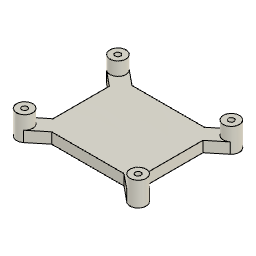
Toolhead Breakout PCB Mount (Autodesk Fusion 360 design; units mm, degrees)
Autodesk Fusion 360 part; units mm, degrees
sketch "Sketch1" plane through (0, 0, 0) normal (0, 0, 1) x (1, 0, 0)
  line L0 (21.185, 17.41) -> (-21.185, 17.41) construction
  line L1 (-21.185, 17.41) -> (-21.185, -17.41) construction
  line L2 (-21.185, -17.41) -> (21.185, -17.41) construction
  line L3 (21.185, -17.41) -> (21.185, 17.41) construction
  line L4 (21.185, 17.41) -> (-21.185, -17.41) construction
  line L5 (-21.185, 17.41) -> (21.185, -17.41) construction
  circle A0 centre (-21.185, 17.41) radius 0.85
  circle A1 centre (-21.185, -17.41) radius 0.85
  circle A2 centre (21.185, -17.41) radius 0.85
  circle A3 centre (21.185, 17.41) radius 0.85
  circle A4 centre (-21.185, 17.41) radius 3
  line L6 (-23.0897, 15.0923) -> (-17.5, 10.4986)
  line L7 (17.5, 15) -> (-17.5, 15)
  line L8 (-17.5, 15) -> (-17.5, -15)
  line L9 (-17.5, -15) -> (17.5, -15)
  line L10 (17.5, -15) -> (17.5, 15)
  line L11 (17.5, 15) -> (-17.5, -15) construction
  line L12 (-17.5, 15) -> (17.5, -15) construction
  line L13 (-13.5274, 15) -> (-19.2803, 19.7277)
  circle A5 centre (21.185, 17.41) radius 3
  circle A6 centre (21.185, -17.41) radius 3
  circle A7 centre (-21.185, -17.41) radius 3
  line L14 (0, 0) -> (0, 14.4635) construction
  line L15 (0, 0) -> (27.8853, 0) construction
  line L16 (23.0897, 15.0923) -> (17.5, 10.4986)
  line L17 (13.5274, 15) -> (19.2803, 19.7277)
  line L18 (-23.0897, -15.0923) -> (-17.5, -10.4986)
  line L19 (-13.5274, -15) -> (-19.2803, -19.7277)
  line L20 (13.5274, -15) -> (19.2803, -19.7277)
  line L21 (23.0897, -15.0923) -> (17.5, -10.4986)
  dimension "d1" = 42.37
  dimension "d2" = 34.82
  dimension "d3" = 1.7
  dimension "d4" = 6
  dimension "d5" = 35
  dimension "d6" = 30
  constraint horizontal L0
  constraint perpendicular L0 L1
  constraint parallel L0 L2
  constraint parallel L1 L3
  constraint coincident L4 L14.start
  constraint coincident L5 L14.start
  constraint coincident L14.start L15.start
  constraint coincident L0.end L1.start
  constraint coincident L1.end L2.start
  constraint coincident L2.end L3.start
  constraint coincident L0.start L3.end
  constraint equal A0 A3
  constraint equal A0 A1
  constraint equal A0 A2
  constraint concentric A0 A4
  constraint coincident A4 L6.start
  constraint parallel L5 L6
  constraint tangent A4 L6
  constraint horizontal L7
  constraint perpendicular L7 L8
  constraint parallel L7 L9
  constraint parallel L8 L10
  constraint coincident L11 L14.start
  constraint coincident L12 L14.start
  constraint parallel L6 L13
  constraint coincident A4 L13.end
  constraint tangent A4 L13
  constraint coincident L7 L13.start
  constraint coincident L6.end L8
  constraint concentric A3 A5
  constraint concentric A2 A6
  constraint concentric A1 A7
  constraint equal A4 A5
  constraint equal A4 A7
  constraint equal A4 A6
  constraint perpendicular L0 L14
  constraint perpendicular L14 L15
  constraint symmetric L6.start L14 L16.start
  constraint symmetric L6.end L14 L16.end
  constraint symmetric L13.start L14 L17.start
  constraint symmetric L13.end L14 L17.end
  constraint symmetric L6.start L15 L18.start
  constraint symmetric L6.end L15 L18.end
  constraint symmetric L13.start L15 L19.start
  constraint symmetric L13.end L15 L19.end
  constraint symmetric L15 L16.start L21.start
  constraint symmetric L15 L16.end L21.end
  constraint symmetric L15 L17.start L20.start
  constraint symmetric L15 L17.end L20.end
  measures "d1" distance of L0.start L0.end
  measures "d2" distance of L0.end L1.end
  measures "d3" diameter of A3
  measures "d4" diameter of A4
  measures "d5" distance of L8.end L9.end
  measures "d6" distance of L7.start L9.end
extrude "Extrude1" add sketch "Sketch1" along normal blind 4
sketch "Sketch2" plane through (0, 0, 4) normal (0, 0, 1) x (-1, 0, 0)
  circle A0 centre (21.185, -17.41) radius 0.85
  circle A1 centre (-21.185, -17.41) radius 0.85
  circle A2 centre (-21.185, 17.41) radius 0.85
  circle A3 centre (21.185, 17.41) radius 0.85
  line L0 (13.5274, 15) -> (-13.5274, 15)
  line L1 (-13.5274, 15) -> (-19.2803, 19.7277)
  arc A4 (-19.2803, 19.7277) -> (-23.0897, 15.0923) centre (-21.185, 17.41) ccw
  line L2 (-23.0897, 15.0923) -> (-17.5, 10.4986)
  line L3 (-17.5, 10.4986) -> (-17.5, -10.4986)
  line L4 (-17.5, -10.4986) -> (-23.0897, -15.0923)
  arc A5 (-23.0897, -15.0923) -> (-19.2803, -19.7277) centre (-21.185, -17.41) ccw
  line L5 (-19.2803, -19.7277) -> (-13.5274, -15)
  line L6 (-13.5274, -15) -> (13.5274, -15)
  line L7 (13.5274, -15) -> (19.2803, -19.7277)
  arc A6 (19.2803, -19.7277) -> (23.0897, -15.0923) centre (21.185, -17.41) ccw
  line L8 (23.0897, -15.0923) -> (17.5, -10.4986)
  line L9 (17.5, -10.4986) -> (17.5, 10.4986)
  line L10 (17.5, 10.4986) -> (23.0897, 15.0923)
  arc A7 (23.0897, 15.0923) -> (19.2803, 19.7277) centre (21.185, 17.41) ccw
  line L11 (19.2803, 19.7277) -> (13.5274, 15)
  circle A8 centre (21.185, -17.41) radius 3
  circle A9 centre (21.185, 17.41) radius 3
  circle A10 centre (-21.185, -17.41) radius 3
  circle A11 centre (-21.185, 17.41) radius 3
  constraint concentric A0 A8
  constraint concentric A3 A9
  constraint tangent L10 A9
  constraint concentric A1 A10
  constraint concentric A2 A11
extrude "Extrude2" add sketch "Sketch2" along normal blind 5 contours A7 A9 | A4 A11 | A6 A8 | A5 A10
sketch "Sketch3" plane through (0, 0, 9) normal (0, 0, 1) x (-1, 0, 0)
  circle A0 centre (21.185, -17.41) radius 0.85
  circle A1 centre (21.185, -17.41) radius 3
  circle A2 centre (-21.185, 17.41) radius 0.85
  circle A3 centre (-21.185, -17.41) radius 0.85
  circle A4 centre (21.185, 17.41) radius 0.85
  circle A5 centre (21.185, -17.41) radius 1.05
  circle A6 centre (-21.185, -17.41) radius 1.05
  circle A7 centre (-21.185, 17.41) radius 1.05
  circle A8 centre (21.185, 17.41) radius 1.05
  dimension "d11" = 2.1
  constraint concentric A0 A5
  constraint concentric A3 A6
  constraint concentric A2 A7
  constraint concentric A4 A8
  constraint equal A5 A6
  constraint equal A6 A8
  constraint equal A7 A8
  measures "d11" diameter of A5
extrude "Extrude3" cut sketch "Sketch3" against normal blind 3 contours A5 | A6 | A7 | A8
